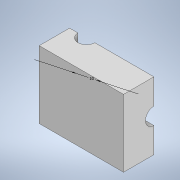
# Autodesk Inventor part: perpendicular connector mould small
Saved by Autodesk Inventor 2022 (Build 260153000, 153)
## iProperties
Created: 2021-09-08
Part Number: perpendicular connector mould small
Material: Generic
Document SubType Name: Modeling
Designer: Ferdinand Hubbard
Density: 1 g/cm^3
Appearance: Default
Author: Ferdinand Hubbard
Autodesk Inventor part; units mm, degrees
ref_plane "YZ Plane" through (0, 0, 0) normal (1, 0, 0) x (0, 1, 0)
ref_plane "XZ Plane" through (0, 0, 0) normal (0, 1, 0) x (-1, 0, 0)
ref_plane "XY Plane" through (0, 0, 0) normal (0, 0, 1) x (1, 0, 0)
sketch "Sketch1" plane through (0, 0, 0) normal (0, 1, 0) x (-1, 0, 0)
  circle A0 centre (0, 0) radius 5
  dimension "d0" = 10
  constraints: 1 centre point, 1 coincident
  measures "d0" diameter of A0
extrude "Extrusion1" add sketch "Sketch1" along normal mid plane 40
sketch "Sketch2" plane through (0, 0, 0) normal (1, 0, 0) x (0, 1, 0)
  circle A0 centre (0, 0) radius 5
  dimension "d3" = 10
  constraints: 1 centre point, 1 coincident
  measures "d3" diameter of A0
extrude "Extrusion2" add sketch "Sketch2" along normal blind 40
split "Split1" plane through (0, 0, 0) removes the side toward (0, 0, -1)
sketch "Sketch3" plane through (40, 5, 0) normal (0, 0, -1) x (-1, 0, 0)
  line L0 (50, 15) -> (0, 15)
  line L1 (0, 15) -> (0, -25)
  line L2 (0, -25) -> (50, -25)
  line L3 (50, -25) -> (50, 15)
  point P0 (40, -5)
  dimension "d6" = 50
  dimension "d7" = 40
  constraints: 8 end point, 2 parallel, 1 horizontal, 1 perpendicular
  measures "d6" distance of L2.end L1.end
  measures "d7" distance of L1.end L0.end
extrude "Extrusion3" add sketch "Sketch3" against normal blind 18 separate body
combine bodies "Combine1" operation type subtract main body 2 bodies to subtract 1
fillet "Fillet1" radius 10 2 edges at (3.5355, -3.5355, 3.5355) (3.5355, 3.5355, 3.5355)
body "Solid2"
